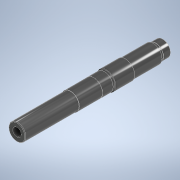
# Autodesk Inventor part: shaft
Saved by Autodesk Inventor 2022 (Build 260153000, 153)
## iProperties
Created: 2025-01-13
Part Number: shaft
Material: Generic
Document SubType Name: Modeling
Designer: Home
Density: 1 g/cm^3
Appearance: Dark Gray
Author: Home
Autodesk Inventor part; units mm, degrees
ref_plane "XZ Plane" through (0, 0, 0) normal (0, 1, 0) x (-1, 0, 0)
ref_plane "XY Plane" through (0, 0, 0) normal (0, 0, 1) x (1, 0, 0)
sketch "Sketch1" plane through (0, 0, 0) normal (0, 0, 1) x (1, 0, 0)
  circle A0 centre (0, 0) radius 7.5
  dimension "d0" = 15
  constraints: 1 centre point, 1 coincident
  measures "d0" diameter of A0
extrude "Extrusion1" add sketch "Sketch1" along normal blind 7
sketch "Sketch2" plane through (0, 0, 7) normal (0, 0, 1) x (1, 0, 0)
  circle A0 centre (0, 0) radius 7.25
  dimension "d3" = 14.5
  constraints: 1 centre point, 1 coincident
  measures "d3" diameter of A0
extrude "Extrusion2" add sketch "Sketch2" along normal blind 2.5
sketch "Sketch3" plane through (0, 0, 9.5) normal (0, 0, 1) x (1, 0, 0)
  circle A0 centre (0, 0) radius 8.5
  dimension "d6" = 17
  constraints: 1 centre point, 1 coincident
  measures "d6" diameter of A0
extrude "Extrusion3" add sketch "Sketch3" along normal blind 44.5
sketch "Sketch4" plane through (0, 0, 54) normal (0, 0, 1) x (1, 0, 0)
  circle A0 centre (0, 0) radius 8.25
  dimension "d9" = 16.5
  constraints: 1 centre point, 1 coincident
  measures "d9" diameter of A0
extrude "Extrusion4" add sketch "Sketch4" along normal blind 2
sketch "Sketch5" plane through (0, 0, 56) normal (0, 0, 1) x (1, 0, 0)
  circle A0 centre (0, 0) radius 8.5
  dimension "d12" = 17
  constraints: 1 centre point, 1 coincident
  measures "d12" diameter of A0
extrude "Extrusion5" add sketch "Sketch5" along normal blind 10
sketch "Sketch6" plane through (0, 0, 66) normal (0, 0, 1) x (1, 0, 0)
  circle A0 centre (0, 0) radius 8.45
  dimension "d15" = 16.9
  constraints: 1 centre point, 1 coincident
  measures "d15" diameter of A0
extrude "Extrusion6" add sketch "Sketch6" along normal blind 22
sketch "Sketch7" plane through (0, 0, 88) normal (0, 0, 1) x (1, 0, 0)
  circle A0 centre (0, 0) radius 8.1
  dimension "d18" = 16.2
  constraints: 1 centre point, 1 coincident
  measures "d18" diameter of A0
extrude "Extrusion7" add sketch "Sketch7" along normal blind 51
sketch "Sketch8" plane through (0, 0, 139) normal (0, 0, 1) x (1, 0, 0)
  line L0 (-5.4, 8.2708) -> (-5.4, -12.4422)
  line L1 (-5.4, -12.4422) -> (-13.0378, -12.4422)
  line L2 (-13.0378, -12.4422) -> (-13.0378, 8.2708)
  line L3 (-13.0378, 8.2708) -> (-5.4, 8.2708)
  point P0 (0, 0)
  dimension "d63" = 5.4
  constraints: 8 end point, 2 parallel, 1 perpendicular, 1 vertical
  measures "d63" distance from line of point (0, 0) L0
extrude "Extrusion8" cut sketch "Sketch8" against normal blind 47.5
sketch "Sketch9" plane through (0, 0, 139) normal (0, 0, 1) x (1, 0, 0)
  arc A0 (-5.4, -6.0374) -> (-5.4, 6.0374) centre (0, 0) ccw projected
  circle A1 centre (0, 0) radius 8.1
  point P0 (-6.0374, 5.4)
  point P1 (6.0374, 5.4)
  point P2 (6.0374, 5.4)
  point P3 (-6.0374, 5.4)
  constraints: 1 coincident, 2 other
extrude "Extrusion9" add sketch "Sketch9" against normal blind 3
sketch "Sketch10" plane through (0, 0, 54) normal (0, 0, 1) x (1, 0, 0)
  circle A0 centre (0, 0) radius 9
  dimension "d26" = 18
  constraints: 1 centre point, 1 coincident
  measures "d26" diameter of A0
extrude "Extrusion10" add sketch "Sketch10" against normal blind 18
chamfer "Chamfer1" distance 0.05 angle 45 1 edges at (-8.45, 0, 66)
ref_plane "Work Plane1" through (-5, 0, 0) normal (1, 0, 0) x (0, 1, 0)
sketch "Sketch11" plane through (-5, 0, 0) normal (1, 0, 0) x (0, 1, 0)
  line L0 (0, 23.5) -> (0, 30.5) construction
  line L1 (2.5, 23.5) -> (2.5, 30.5)
  line L2 (-2.5, 30.5) -> (-2.5, 23.5)
  arc A0 (-2.5, 23.5) -> (2.5, 23.5) centre (0, 23.5) ccw
  arc A1 (2.5, 30.5) -> (-2.5, 30.5) centre (0, 30.5) ccw
  line L3 (7.5, 0) -> (-7.5, 0) projected
  point P0 (0, 0)
  point P1 (0, 27)
  dimension "d33" = 7
  dimension "d34" = 5
  dimension "d35" = 0
  dimension "d36" = 23.5
  constraints: 8 end point, 4 point on circle, 4 tangent, 2 centre point, 1 midpoint, 1 parallel, 1 vertical
  measures "d33" distance of L0.start L0.end
  measures "d34" diameter of A1
  measures "d35" horizontal distance of point (0, 0) point (0, 27)
  measures "d36" distance from line of L3 L0.start
extrude "Extrusion11" cut sketch "Sketch11" against normal blind 22
chamfer "Chamfer2" distance 0.5 angle 45 2 edges at (-7.5, 0, 0) (-8.1, 0, 139)
sketch "Sketch12" plane through (0, 0, 0) normal (0, 1, 0) x (-1, 0, 0)
  line L0 (9, 54) -> (9, 36) projected
  line L1 (9, 43) -> (1.9289, 50.0711)
  line L2 (1.9289, 50.0711) -> (6.1716, 54.3137)
  line L3 (6.1716, 54.3137) -> (13.2426, 47.2426)
  line L4 (13.2426, 47.2426) -> (9, 43)
  line L5 (9, 43) -> (19, 43) construction
  line L6 (-9, 36) -> (9, 36) projected
  point P0 (0, 0)
  dimension "d42" = 10
  dimension "d43" = 135
  dimension "d44" = 6
  dimension "d47" = 7
  constraints: 10 end point, 2 parallel, 1 equal length, 1 horizontal, 1 perpendicular, 1 point on line
  measures "d42" distance of L1.start L1.end
  measures "d43" angle of L5 L1
  measures "d44" distance of L3.end L1.start
  measures "d47" distance from line of L6 L1.start
extrude "Extrusion12" cut sketch "Sketch12" along normal mid plane 6
fillet "Fillet1" radius 3 4 edges at (-7.3284, -3, 53.1569) (-5.2071, 3, 46.7929) (-5.2071, -3, 46.7929) (-7.3284, 3, 53.1569)
sketch "Sketch13" plane through (0, 0, 139) normal (0, 0, 1) x (1, 0, 0)
  circle A0 centre (0, 0) radius 8.1 projected
  constraints: 1 coincident
hole "Hole1" at (0, 0, 139) direction (0, 0, -1) diameter 8 depth 96 tip angle 118
sketch "Sketch14" plane through (-4.0503, 0, 52.1924) normal (-0.7071068, 0, -0.7071068) x (-0.7071068, 0, 0.7071068)
  arc A0 (-1.4567, -2.6226) -> (-1.4567, 2.6226) centre (0, 0) ccw projected
  point P0 (-39.7696, 0)
  constraints: 1 coincident
hole "Hole2" at (-4.0503, 0, 52.1924) direction (0.7071068, 0, 0.7071068) diameter 6 depth 4.75 tip angle 118
body "Solid1"
